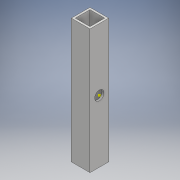
# Autodesk Inventor part: Pipe3
Saved by Autodesk Inventor 2018 (Build 220112000, 112)
## iProperties
Created: 2017-09-10
Part Number: Pipe3
Material: 一般
Document SubType Name: Modeling
Designer: mura5
Density: 1 g/cm^3
Appearance: 既定
Author: mura5
Autodesk Inventor part; units mm, degrees
ref_plane "YZ Plane" through (0, 0, 0) normal (1, 0, 0) x (0, 1, 0)
ref_plane "XZ Plane" through (0, 0, 0) normal (0, 1, 0) x (-1, 0, 0)
ref_plane "XY Plane" through (0, 0, 0) normal (0, 0, 1) x (1, 0, 0)
sketch "スケッチ1" plane through (0, 0, 0) normal (0, 0, 1) x (1, 0, 0)
  line L0 (15, -15) -> (-15, -15)
  line L1 (-15, -15) -> (-15, 15)
  line L2 (-15, 15) -> (15, 15)
  line L3 (15, 15) -> (15, -15)
  line L4 (15, -15) -> (-15, 15) construction
  line L5 (-15, -15) -> (15, 15) construction
  line L6 (11.8, 11.8) -> (-11.8, 11.8)
  line L7 (-11.8, 11.8) -> (-11.8, -11.8)
  line L8 (-11.8, -11.8) -> (11.8, -11.8)
  line L9 (11.8, -11.8) -> (11.8, 11.8)
  point P0 (0, 0)
  dimension "d0" = 30
  dimension "d1" = 30
  dimension "d2" = 3.2
  constraints: 20 end point, 4 parallel, 2 midpoint, 2 perpendicular, 1 horizontal, 3 other
  measures "d0" distance of L1.end L2.end
  measures "d1" distance of L0.end L1.end
  measures "d2" distance between parallel lines of L2 L6
extrude "押し出し1" add sketch "スケッチ1" along normal mid plane 200
sketch "スケッチ2" plane through (15, -15, -100) normal (1, 0, 0) x (0, 0, -1)
  point P0 (-100, 15)
sketch "スケッチ3" plane through (15, -15, 100) normal (1, 0, 0) x (0, 0, -1)
  circle A0 centre (100, 15) radius 7.5
  dimension "d7" = 15
  constraints: 1 centre point, 1 coincident
  measures "d7" diameter of A0
extrude "押し出し2" cut sketch "スケッチ3" against normal blind 30
